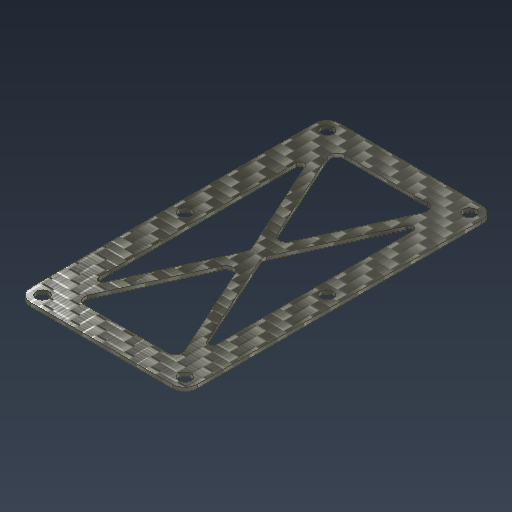
# Autodesk Inventor part: Tattu_Battery__Top_Tray
Saved by Autodesk Inventor 2024.1 (Build 281209000, 209)
## iProperties
Created: 2023-06-26
Part Number: Tattu_Battery__Top_Tray
Material: CFRP
Document SubType Name: Modeling
Designer: dzw04
Density: 1.43 g/cm^3
Appearance: Carbon Fiber 1
Mass: 3.00573 g
Surface Area: 49.6467 cm^2
Volume: 2.10191 cm^3
Author: dzw04
Autodesk Inventor part; units mm, degrees
ref_plane "YZ Plane" through (0, 0, 0) normal (1, 0, 0) x (0, 1, 0)
ref_plane "XZ Plane" through (0, 0, 0) normal (0, 1, 0) x (-1, 0, 0)
ref_plane "XY Plane" through (0, 0, 0) normal (0, 0, 1) x (1, 0, 0)
sketch "Sketch1" plane through (0, 0, 0) normal (0, 1, 0) x (-1, 0, 0)
  line L0 (-20, 40) -> (20, 40) construction
  line L1 (20, 40) -> (20, -40) construction
  line L2 (20, -40) -> (-20, -40) construction
  line L3 (-20, -40) -> (-20, 40) construction
  line L4 (-20, 40) -> (20, -40) construction
  line L5 (20, 40) -> (-20, -40) construction
  circle A0 centre (20, 40) radius 1.75
  circle A1 centre (20, -40) radius 1.75
  circle A2 centre (-20, -40) radius 1.75
  circle A3 centre (-20, 40) radius 1.75
  circle A4 centre (20, 0) radius 1.75
  circle A5 centre (-20, 0) radius 1.75
  line L6 (-20, 43.5) -> (20, 43.5)
  line L7 (23.5, 40) -> (23.5, -40)
  line L8 (20, -43.5) -> (-20, -43.5)
  line L9 (-23.5, -40) -> (-23.5, 40)
  line L10 (-23.5, 43.5) -> (23.5, -43.5) construction
  line L11 (23.5, 43.5) -> (-23.5, -43.5) construction
  arc A6 (23.5, 40) -> (20, 43.5) centre (20, 40) ccw
  arc A7 (-20, 43.5) -> (-23.5, 40) centre (-20, 40) ccw
  arc A8 (-23.5, -40) -> (-20, -43.5) centre (-20, -40) ccw
  arc A9 (20, -43.5) -> (23.5, -40) centre (20, -40) ccw
  point P0 (0, 0)
  dimension "d0" = 40
  dimension "d1" = 80
  dimension "d2" = 3.5
  dimension "d3" = 3.5
  dimension "d4" = 3.5
  dimension "d5" = 3.5
  dimension "d6" = 3.5
  dimension "d7" = 3.5
  dimension "d8" = 47
  dimension "d9" = 87
  dimension "d10" = 3.5
  constraints: 24 end point, 10 centre point, 8 point on circle, 8 point on line, 8 tangent, 6 midpoint, 4 coincident, 4 parallel, 3 equal radius, 2 horizontal, 2 perpendicular
  measures "d0" distance of L1.end L2.end
  measures "d1" distance of L0.end L1.end
  measures "d2" diameter of A0
  measures "d3" diameter of A1
  measures "d4" diameter of A2
  measures "d5" diameter of A3
  measures "d6" diameter of A4
  measures "d7" diameter of A5
  measures "d8" distance of L10.end L11.end
  measures "d9" distance of L11.start L10.end
  measures "d10" radius of A6
extrude "Extrusion1" add sketch "Sketch1" along normal blind 1
sketch "Sketch2" plane through (0, 1, 0) normal (0, 1, 0) x (1, 0, 0)
  line L0 (-16.5, -36.5) -> (16.5, -36.5)
  line L1 (16.5, -36.5) -> (16.5, 36.5)
  line L2 (16.5, 36.5) -> (-16.5, 36.5)
  line L3 (-16.5, 36.5) -> (-16.5, -36.5)
  line L4 (-16.5, -36.5) -> (16.5, 36.5)
  line L5 (16.5, -36.5) -> (-16.5, 36.5)
  line L6 (15.1332, -37.1179) -> (-17.8668, 35.8821)
  line L7 (17.8668, -35.8821) -> (-15.1332, 37.1179)
  line L8 (-17.8668, -35.8821) -> (15.1332, 37.1179)
  line L9 (-15.1332, -37.1179) -> (17.8668, 35.8821)
  point P0 (0, 0)
  point P1 (16.5, 32.8585)
  point P2 (1.6461, 0)
  point P3 (16.5, -32.8585)
  point P4 (0, 3.6415)
  point P5 (14.8539, 36.5)
  point P6 (-14.8539, 36.5)
  point P7 (0, -3.6415)
  point P8 (-14.8539, -36.5)
  point P9 (14.8539, -36.5)
  point P10 (-16.5, -32.8585)
  point P11 (-1.6461, 0)
  point P12 (-16.5, 32.8585)
  dimension "d13" = 33
  dimension "d14" = 73
  dimension "d15" = 1.5
  dimension "d16" = 1.5
  dimension "d17" = 1.5
  dimension "d18" = 1.5
  constraints: 20 end point, 6 parallel, 2 midpoint, 1 horizontal, 1 perpendicular
  measures "d13" distance of L2.end L1.end
  measures "d14" distance of L1.end L0.end
  measures "d15" distance between parallel lines of L5 L6
  measures "d16" distance between parallel lines of L5 L7
  measures "d17" distance between parallel lines of L4 L8
  measures "d18" distance between parallel lines of L4 L9
extrude "Extrusion2" cut sketch "Sketch2" against normal through all contours L9 L6 L0 | L3 L6 L8 | L7 L9 L1 | L2 L8 L7
fillet "Fillet1" radius 2 8 edges at (-14.8539, 0.5, 36.5) (14.8539, 0.5, 36.5) (-14.8539, 0.5, -36.5) (14.8539, 0.5, -36.5) (1.6461, 0.5, 0) (-1.6461, 0.5, 0) (0, 0.5, 3.6415) (0, 0.5, -3.6415)
fillet "Fillet2" radius 1.1 4 edges at (16.5, 0.5, 32.8585) (-16.5, 0.5, 32.8585) (-16.5, 0.5, -32.8585) (16.5, 0.5, -32.8585)
equation "\"d11\" = ThicknessBatteryTopTray"
equation "\"MountToMotorCenter\" = 0"
equation "\"ArmPosition\" = 5deg"
equation "\"BatteryWidth\" = 62"
equation "\"BatteryHeight\" = 76"
equation "\"ThicknessBodyOuterPlate\" = 2"
equation "\"ThicknessBodyCenterPlate\" = 2"
equation "\"ThicknessLegLoadpipePlate\" = 2"
equation "\"ThicknessBatteryTray\" = 2"
equation "\"ThicknessBatteryTopTray\" = 1"
equation "\"LandingGearStabilityBar\" = 525"
equation "\"StartAngleArm\" = 45deg"
equation "\"MotorMountCenter\" = 71.5"
body "Solid1"
